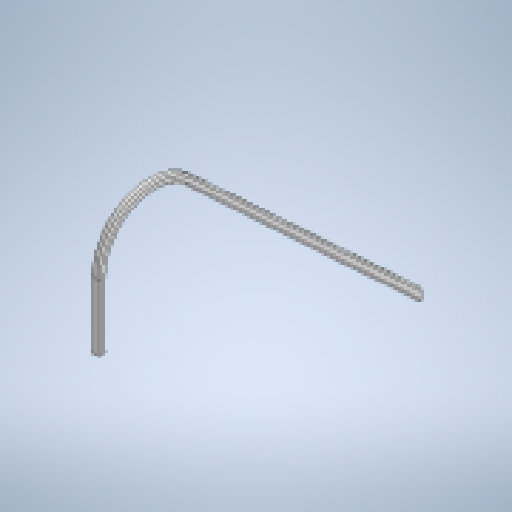
# Autodesk Inventor part: cable
Saved by Autodesk Inventor 2025.2 (Build 292293000, 293)
## iProperties
Created: 2025-08-19
Part Number: cable
Material: 一般
Document SubType Name: Modeling
Designer: naka6
Density: 1 g/cm^3
Appearance: 既定
Author: naka6
Autodesk Inventor part; units mm, degrees
ref_plane "YZ Plane" through (0, 0, 0) normal (1, 0, 0) x (0, 1, 0)
ref_plane "XZ Plane" through (0, 0, 0) normal (0, 1, 0) x (-1, 0, 0)
ref_plane "XY Plane" through (0, 0, 0) normal (0, 0, 1) x (1, 0, 0)
sketch "スケッチ1" plane through (0, 0, 0) normal (1, 0, 0) x (0, 1, 0)
  line L0 (-29.160648, 22.602351) -> (-26.160648, 22.602351)
  line L1 (-26.160648, 22.102351) -> (-29.160648, 22.102351)
  spline S0 degree 3 poles (-39.675758, -20.959231) (-39.675746, -19.525228) (-39.67573, -18.187156) (-39.67571, -16.984398) knots 0 0 0 0 1 1 1 1
  ellipse E0 centre (-39.675628, -20.058524) end of major axis (-39.675628, -15.058524) minor radius 0.000104 (-39.675628, -15.058524) -> (-39.67571, -16.984399) ccw
  line L2 (-39.675623, -16.058524) -> (-38.075623, -16.058524)
  line L3 (-38.075623, -16.058524) -> (-38.075623, -36.058524)
  line L4 (-26.160648, 22.102351) -> (-18.111397, 22.102351)
  arc A0 (-13.3776, 12.543762) -> (-18.111397, 22.102351) centre (-18.111397, 16.150874) ccw
  line L5 (-13.3776, 12.543762) -> (-43.581994, -19.874933)
  line L6 (-43.581994, -19.874933) -> (-13.3776, 12.543762)
  arc A1 (-43.581994, -19.874933) -> (-39.67571, -16.984399) centre (-33.849641, -28.942535) ccw
  arc A2 (-12.582202, 11.937675) -> (-18.111397, 23.102351) centre (-18.111397, 16.150874) ccw
  line L7 (-18.111397, 23.102351) -> (-26.160648, 23.102351)
  line L8 (-26.160648, 23.102351) -> (-29.160648, 23.102351)
  arc A3 (-41.637103, -19.419312) -> (-40.675728, -18.708236) centre (-33.849641, -28.942535) ccw
  line L9 (-12.582202, 11.937675) -> (-41.637103, -19.419312)
  line L10 (-26.160648, 23.102351) -> (-26.160648, 22.102351)
  line L11 (-38.075623, -16.058524) -> (-40.026258, -16.058524)
  point P0 (0, 0)
  point P1 (-38.675679, -15.048445)
  point P2 (-38.675758, -20.959239)
  point P3 (-40.405833, -16.058524)
  point P4 (-38.675603, -16.058524)
  point P5 (-39.675715, -17.302519)
  point P6 (-39.67571, -16.984398)
  point P7 (-39.675679, -15.682243)
  point P8 (-38.075623, -16.329796)
  point P9 (-38.075623, -17.389292)
  point P10 (-39.161062, -16.747089)
  point P11 (-39.67571, -16.984399)
  point P12 (-38.675698, -16.223268)
  point P13 (-38.523048, -16.058524)
  point P14 (-38.675695, -16.058524)
  point P15 (-39.675727, -18.107727)
  point P16 (-38.67572, -17.626825)
  point P17 (-38.675703, -16.547002)
  dimension "d0" = 1
  dimension "d1" = 1
  constraints: 16 end point, 8 point on circle, 4 centre point, 2 point on line, 2 tangent, 1 collinear, 1 concentric, 1 horizontal, 1 vertical, 9 other
  measures "d0" radial gap between concentric circles of A0 A2
  measures "d1" radial gap between concentric circles of A1 A3
extrude "押し出し1" add sketch "スケッチ1" along normal blind 1 contours L11 L5 E0 | E0 L5 A0 L4 L10 L7 A2 L9 L2
fillet "フィレット1" radius 0.25 12 edges at (1, -25.5526, -2.0604) (1, -26.7019, -1.7574) (0, -25.5526, -2.0604) (1, -22.136, 23.1024) (1, -11.882, 19.2359) (0, -22.136, 23.1024) (0, -11.882, 19.2359) (1, -22.136, 22.1024) (1, -12.7781, 18.7921) (0, -22.136, 22.1024) (0, -12.7781, 18.7921) (0, -26.7019, -1.7574)
